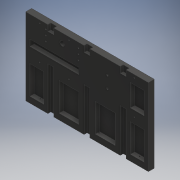
# Autodesk Inventor part: HB03
Saved by Autodesk Inventor 2017 (Build 210142000, 142)
## iProperties
Created: 2019-05-20
Part Number: HB03
Material: Polyethylene, High Density
Document SubType Name: Modeling
Designer: Dell
Density: 0.952 g/cm^3
Appearance: Smooth - Black
Mass: 3129.5 g
Surface Area: 4619.69 cm^2
Volume: 3287.29 cm^3
Author: Dell
Autodesk Inventor part; units mm, degrees
ref_plane "YZ Plane" through (0, 0, 0) normal (1, 0, 0) x (0, 1, 0)
ref_plane "XZ Plane" through (0, 0, 0) normal (0, 1, 0) x (-1, 0, 0)
ref_plane "XY Plane" through (0, 0, 0) normal (0, 0, 1) x (1, 0, 0)
sketch "Sketch1" plane through (0, 0, 0) normal (0, 0, 1) x (1, 0, 0)
  line L0 (0, 0) -> (525.78, 0)
  line L1 (525.78, 0) -> (525.78, 25.4)
  line L2 (525.78, 25.4) -> (0, 25.4)
  line L3 (0, 25.4) -> (0, 0)
  dimension "d0" = 525.78
  dimension "d1" = 25.4
  constraints: 8 end point, 2 parallel, 1 horizontal, 1 perpendicular
  measures "d0" distance of L2.end L1.end
  measures "d1" distance of L1.end L0.end
extrude "Extrusion1" add sketch "Sketch1" along normal blind 330.2
sketch "Sketch3" plane through (0, 25.4, 0) normal (0, 1, 0) x (1, 0, 0)
  line L0 (0, -330.2) -> (525.78, -330.2) construction
  line L1 (525.78, -330.2) -> (525.78, -241.3)
  line L2 (525.78, -241.3) -> (0, -241.3) construction
  line L3 (0, -241.3) -> (0, -330.2) construction
  line L4 (86.36, -308.25) -> (86.36, -263.25) construction
  circle A0 centre (86.36, -285.75) radius 2.3812
  circle A1 centre (86.36, -308.25) radius 2.3812
  circle A2 centre (86.36, -263.25) radius 2.3812
  line L5 (146.36, -280.75) -> (146.36, -300.75) construction
  line L6 (156.36, -263.25) -> (156.36, -308.25) construction
  line L7 (146.36, -300.75) -> (166.36, -300.75) construction
  line L8 (166.36, -280.75) -> (146.36, -280.75) construction
  line L9 (86.36, -263.25) -> (226.36, -263.25) construction
  line L10 (226.36, -308.25) -> (86.36, -308.25) construction
  line L11 (86.36, -285.75) -> (226.36, -285.75) construction
  line L12 (166.36, -300.75) -> (166.36, -280.75) construction
  line L13 (226.36, -263.25) -> (226.36, -308.25) construction
  circle A3 centre (226.36, -263.25) radius 2.3813
  circle A4 centre (226.36, -285.75) radius 2.3813
  circle A5 centre (226.36, -308.25) radius 2.3813
  circle A6 centre (156.36, -290.75) radius 10
  line L14 (0, 0) -> (0, -330.2) projected
  point P0 (525.78, 0)
  point P1 (0, -285.75)
  point P2 (146.36, -290.75)
  point P3 (166.36, -290.75)
  dimension "d16" = 45
  dimension "d17" = 140
  dimension "d18" = 4.7625
  dimension "d19" = 4.7625
  dimension "d20" = 4.7625
  dimension "d21" = 4.7625
  dimension "d22" = 4.7625
  dimension "d23" = 4.7625
  dimension "d24" = 60
  dimension "d25" = 7.5
  dimension "d26" = 20
  dimension "d27" = 20
  dimension "d28" = 86.36
  dimension "d29" = 88.9
  constraints: 28 end point, 7 midpoint, 6 centre point, 6 parallel, 5 coincident, 3 horizontal alignment, 3 perpendicular, 2 point on line, 1 horizontal, 2 other
  measures "d16" distance of L13.start L13.end
  measures "d17" distance of L9.start L13.start
  measures "d18" diameter of A2
  measures "d19" diameter of A0
  measures "d20" diameter of A1
  measures "d21" diameter of A5
  measures "d22" diameter of A4
  measures "d23" diameter of A3
  measures "d24" distance from line of L11.end L12
  measures "d25" distance between parallel lines of L10 L7
  measures "d26" distance of L12.end L8.end
  measures "d27" distance of L8.end L7.start
  measures "d28" distance between parallel lines of L3 L4
  measures "d29" distance of L2.end L0.start
extrude "Extrusion3" cut sketch "Sketch3" against normal through all
sketch "Sketch6" plane through (0, 0, 0) normal (0, 0, -1) x (-1, 0, 0)
  line L0 (0, 0) -> (-525.78, 0) projected
  line L1 (0, 0) -> (-525.78, 0) projected
  line L2 (-275.59, 0) -> (-250.19, 0)
  line L3 (-250.19, 0) -> (-250.19, 12.7)
  line L4 (-250.19, 12.7) -> (-275.59, 12.7)
  line L5 (-275.59, 12.7) -> (-275.59, 0)
  line L6 (-430.79, 0) -> (-405.39, 0)
  line L7 (-405.39, 0) -> (-405.39, 12.7)
  line L8 (-405.39, 12.7) -> (-430.79, 12.7)
  line L9 (-430.79, 12.7) -> (-430.79, 0)
  line L10 (-120.39, 0) -> (-94.99, 0)
  line L11 (-94.99, 0) -> (-94.99, 12.7)
  line L12 (-94.99, 12.7) -> (-120.39, 12.7)
  line L13 (-120.39, 12.7) -> (-120.39, 0)
  line L14 (-120.39, 6.35) -> (-405.39, 6.35)
  point P0 (-262.89, 0)
  point P1 (-94.99, 6.35)
  point P2 (-262.89, 6.35)
  point P3 (-262.89, 0)
  dimension "d34" = 25.4
  dimension "d35" = 12.7
  dimension "d36" = 25.4
  dimension "d37" = 12.7
  dimension "d40" = 25.4
  dimension "d41" = 12.7
  dimension "d47" = 285
  constraints: 26 end point, 7 midpoint, 7 parallel, 3 horizontal, 3 perpendicular, 3 point on line, 1 horizontal alignment, 1 vertical alignment
  measures "d34" distance of L4.end L3.end
  measures "d35" distance of L3.end L2.end
  measures "d36" distance of L8.end L7.end
  measures "d37" distance of L7.end L6.end
  measures "d40" distance of L11.end L12.end
  measures "d41" distance of L10.end L11.end
  measures "d47" distance of L14.start L14.end
extrude "Extrusion5" cut sketch "Sketch6" against normal blind 185 contours L0 L13 L12 L11 | L0 L5 L14 L3 | L14 L5 L4 L3 | L0 L9 L8 L7
sketch "Sketch8" plane through (0, 0, 330.2) normal (0, 0, 1) x (1, 0, 0)
  line L0 (94.99, 0) -> (120.39, 0) projected
  line L1 (94.99, 12.7) -> (94.99, 0) projected
  line L2 (120.39, 12.7) -> (94.99, 12.7) projected
  line L3 (120.39, 0) -> (120.39, 12.7) projected
  line L4 (250.19, 0) -> (275.59, 0) projected
  line L5 (250.19, 12.7) -> (250.19, 0) projected
  line L6 (275.59, 12.7) -> (250.19, 12.7) projected
  line L7 (275.59, 0) -> (275.59, 12.7) projected
  line L8 (405.39, 0) -> (430.79, 0) projected
  line L9 (405.39, 12.7) -> (405.39, 0) projected
  line L10 (430.79, 12.7) -> (405.39, 12.7) projected
  line L11 (430.79, 0) -> (430.79, 12.7) projected
  point P0 (0, 0)
extrude "Extrusion6" cut sketch "Sketch8" against normal blind 25.4
sketch "Sketch11" plane through (0, 0, 0) normal (0, -1, 0) x (1, 0, 0)
  circle A0 centre (60.195, 317.5) radius 2
  circle A1 centre (185.29, 317.5) radius 2
  circle A2 centre (340.49, 317.5) radius 2
  circle A3 centre (465.585, 317.5) radius 2
  circle A4 centre (465.585, 172.3) radius 2
  circle A5 centre (340.49, 172.3) radius 2
  circle A6 centre (185.29, 172.3) radius 2
  circle A7 centre (60.195, 172.3) radius 2
  line L0 (0, 330.2) -> (94.99, 330.2) projected
  line L1 (120.39, 330.2) -> (250.19, 330.2) projected
  line L2 (275.59, 330.2) -> (405.39, 330.2) projected
  line L3 (430.79, 330.2) -> (525.78, 330.2) projected
  line L4 (120.39, 304.8) -> (94.99, 304.8) projected
  line L5 (94.99, 185) -> (120.39, 185) projected
  point P0 (0, 0)
  point P1 (185.29, 330.2)
  point P2 (340.49, 330.2)
  dimension "d57" = 4
  dimension "d58" = 4
  dimension "d59" = 4
  dimension "d60" = 4
  dimension "d61" = 4
  dimension "d62" = 4
  dimension "d63" = 4
  dimension "d64" = 4
  dimension "d65" = 12.7
  dimension "d66" = 12.7
  dimension "d69" = 60.195
  dimension "d70" = 60.195
  constraints: 8 centre point, 6 horizontal alignment, 6 vertical alignment, 2 midpoint
  measures "d57" diameter of A0
  measures "d58" diameter of A1
  measures "d59" diameter of A2
  measures "d60" diameter of A3
  measures "d61" diameter of A4
  measures "d62" diameter of A5
  measures "d63" diameter of A6
  measures "d64" diameter of A7
  measures "d65" distance from line of A0.centre L4
  measures "d66" distance from line of L5 A7.centre
  measures "d69" horizontal distance of L0.start A0.centre
  measures "d70" horizontal distance of L3.end A3.centre
extrude "Extrusion8" cut sketch "Sketch11" against normal through all contours A0 | A1 | A3 | A4 | A6 | A7
sketch "Sketch12" plane through (0, 25.4, 0) normal (0, 1, 0) x (1, 0, 0)
  circle A0 centre (60.195, -172.3) radius 2 projected
  circle A1 centre (185.29, -172.3) radius 2 projected
  circle A2 centre (465.585, -172.3) radius 2 projected
  circle A3 centre (465.585, -317.5) radius 2 projected
  circle A4 centre (185.29, -317.5) radius 2 projected
  circle A5 centre (60.195, -317.5) radius 2 projected
  circle A6 centre (60.195, -172.3) radius 2 projected
  circle A7 centre (60.195, -172.3) radius 6.5
  circle A8 centre (60.195, -317.5) radius 2 projected
  circle A9 centre (60.195, -317.5) radius 6.5
  circle A10 centre (185.29, -317.5) radius 2 projected
  circle A11 centre (185.29, -317.5) radius 6.5
  circle A12 centre (185.29, -172.3) radius 2 projected
  circle A13 centre (185.29, -172.3) radius 6.5
  circle A14 centre (465.585, -317.5) radius 6.5
  circle A15 centre (465.585, -172.3) radius 2 projected
  circle A16 centre (465.585, -172.3) radius 6.5
  point P0 (0, 0)
  dimension "d71" = 13
  dimension "d72" = 13
  dimension "d73" = 13
  dimension "d74" = 13
  dimension "d75" = 13
  dimension "d76" = 13
  constraints: 6 centre point, 6 coincident
  measures "d71" diameter of A7
  measures "d72" diameter of A9
  measures "d73" diameter of A11
  measures "d74" diameter of A13
  measures "d75" diameter of A14
  measures "d76" diameter of A16
extrude "Extrusion9" cut sketch "Sketch12" against normal blind 12.7 contours A0 | A1 | A2 | A3 | A4 | A5 | A7 | A9 | A11 | A13 | A14 | A16
sketch "Sketch13" plane through (0, 25.4, 0) normal (0, 1, 0) x (1, 0, 0)
  circle A0 centre (349.98, -219.9) radius 4
  circle A1 centre (349.98, -269.9) radius 4
  line L0 (525.78, 0) -> (525.78, -330.2) projected
  line L1 (525.78, -330.2) -> (0, -330.2) projected
  point P0 (0, 0)
  dimension "d86" = 8
  dimension "d87" = 8
  dimension "d88" = 175.8
  dimension "d89" = 60.3
  dimension "d90" = 50
  constraints: 2 centre point, 1 vertical alignment
  measures "d86" diameter of A1
  measures "d87" diameter of A0
  measures "d88" distance from line of L0 A1.centre
  measures "d89" distance from line of L1 A1.centre
  measures "d90" distance of A1.centre A0.centre
extrude "Extrusion10" cut sketch "Sketch13" against normal through all
sketch "Sketch14" plane through (0, 25.4, 0) normal (0, 1, 0) x (1, 0, 0)
  circle A0 centre (349.98, -219.9) radius 4 projected
  circle A1 centre (349.98, -269.9) radius 4 projected
  circle A2 centre (349.98, -219.9) radius 7.5
  circle A3 centre (349.98, -269.9) radius 7.5
  point P0 (0, 0)
  dimension "d93" = 15
  dimension "d94" = 15
  constraints: 2 centre point, 2 coincident
  measures "d93" diameter of A2
  measures "d94" diameter of A3
extrude "Extrusion11" cut sketch "Sketch14" against normal blind 12.7 contours A0 | A1 | A2 | A3
sketch "Sketch9" plane through (0, 0, 0) normal (0, -1, 0) x (1, 0, 0)
  line L0 (297.99, 146.9) -> (382.99, 146.9)
  line L1 (382.99, 146.9) -> (382.99, 25.4)
  line L2 (382.99, 25.4) -> (297.99, 25.4)
  line L3 (297.99, 25.4) -> (297.99, 146.9)
  line L4 (448.285, 25.4) -> (508.285, 25.4)
  line L5 (508.285, 25.4) -> (508.285, 146.9)
  line L6 (508.285, 146.9) -> (448.285, 146.9)
  line L7 (448.285, 146.9) -> (448.285, 25.4)
  line L8 (142.79, 25.4) -> (227.79, 25.4)
  line L9 (227.79, 25.4) -> (227.79, 146.9)
  line L10 (227.79, 146.9) -> (142.79, 146.9)
  line L11 (142.79, 146.9) -> (142.79, 25.4)
  line L12 (17.495, 25.4) -> (77.495, 25.4)
  line L13 (77.495, 25.4) -> (77.495, 146.9)
  line L14 (77.495, 146.9) -> (17.495, 146.9)
  line L15 (17.495, 146.9) -> (17.495, 25.4)
  line L16 (430.79, 330.2) -> (525.78, 330.2) projected
  line L17 (275.59, 330.2) -> (405.39, 330.2) projected
  line L18 (120.39, 0) -> (250.19, 0) projected
  line L19 (0, 0) -> (94.99, 0) projected
  line L20 (430.79, 0) -> (525.78, 0) projected
  circle A0 centre (86.36, 263.25) radius 2.3812 projected
  circle A1 centre (465.585, 172.3) radius 2 construction
  circle A2 centre (465.585, 317.5) radius 2 construction
  line L21 (508.285, 197.7) -> (448.285, 197.7)
  line L22 (448.285, 197.7) -> (448.285, 292.1)
  line L23 (448.285, 292.1) -> (508.285, 292.1)
  line L24 (508.285, 292.1) -> (508.285, 197.7)
  line L25 (382.99, 146.9) -> (297.99, 146.9)
  line L26 (297.99, 146.9) -> (297.99, 292.1)
  line L27 (297.99, 292.1) -> (382.99, 292.1)
  line L28 (382.99, 292.1) -> (382.99, 146.9)
  line L29 (227.79, 210.4) -> (17.495, 210.4)
  line L30 (17.495, 210.4) -> (17.495, 237.85)
  line L31 (17.495, 237.85) -> (227.79, 237.85)
  line L32 (227.79, 237.85) -> (227.79, 210.4)
  line L33 (94.99, 185) -> (120.39, 185) projected
  line L34 (448.285, 210.4) -> (382.99, 210.4)
  line L35 (382.99, 210.4) -> (382.99, 279.4)
  line L36 (382.99, 279.4) -> (448.285, 279.4)
  line L37 (448.285, 279.4) -> (448.285, 210.4)
  line L38 (430.79, 185) -> (405.39, 185) projected
  line L39 (405.39, 304.8) -> (430.79, 304.8) projected
  line L40 (227.79, 210.4) -> (297.99, 210.4)
  line L41 (297.99, 210.4) -> (297.99, 237.85)
  line L42 (297.99, 237.85) -> (227.79, 237.85)
  line L43 (227.79, 237.85) -> (227.79, 210.4)
  point P0 (478.285, 146.9)
  point P1 (478.285, 330.2)
  point P2 (340.49, 146.9)
  point P3 (340.49, 330.2)
  point P4 (185.29, 25.4)
  point P5 (185.29, 0)
  point P6 (47.495, 25.4)
  point P7 (47.495, 0)
  dimension "d48" = 60
  dimension "d49" = 60
  dimension "d50" = 85
  dimension "d51" = 85
  dimension "d53" = 25.4
  dimension "d79" = 25.4
  dimension "d80" = 25.4
  dimension "d81" = 25.4
  dimension "d82" = 25.4
  dimension "d83" = 25.4
  dimension "d84" = 25.4
  dimension "d85" = 25.4
  constraints: 72 end point, 18 parallel, 9 horizontal, 9 perpendicular, 9 point on line, 8 midpoint, 8 vertical alignment, 7 horizontal alignment, 2 coincident
  measures "d48" distance of L12.start L12.end
  measures "d49" distance of L4.start L4.end
  measures "d50" distance of L8.start L8.end
  measures "d51" distance of L1.end L2.end
  measures "d53" distance between parallel lines of L20 L4
  measures "d79" distance from line of L6 A1.centre
  measures "d80" distance between parallel lines of L33 L29
  measures "d81" distance from line of A0.centre L31
  measures "d82" distance from line of A1.centre L21
  measures "d83" distance from line of A2.centre L23
  measures "d84" distance between parallel lines of L38 L34
  measures "d85" distance between parallel lines of L39 L36
extrude "Extrusion7" cut sketch "Sketch9" against normal blind 19.05 contours L0 L1 L2 L3 | L29 L30 L31 L32 | L22 L23 L24 L21 | L7 L6 L5 L4 | L11 L10 L9 L8 | L15 L14 L13 L12 | A0
sketch "Sketch15" plane through (0, 0, 0) normal (0, 0, -1) x (-1, 0, 0)
  circle A0 centre (-137.795, 12.7) radius 2
  circle A1 centre (-224.3975, 12.7) radius 2
  line L0 (0, 25.4) -> (0, 0) projected
  line L1 (-525.78, 25.4) -> (0, 25.4) projected
  line L2 (-262.89, 25.4) -> (-262.89, -36.2644)
  circle A2 centre (-387.985, 12.7) radius 2
  circle A3 centre (-301.3825, 12.7) radius 2
  point P0 (0, 12.7)
  dimension "d97" = 4
  dimension "d98" = 4
  dimension "d99" = 86.6025
  dimension "d100" = 137.795
  constraints: 4 centre point, 2 end point, 2 horizontal alignment, 2 midpoint, 2 symmetric about line, 1 vertical, 2 other
  measures "d97" diameter of A0
  measures "d98" diameter of A1
  measures "d99" distance of A0.centre A1.centre
  measures "d100" distance from line of L0 A0.centre
extrude "Extrusion12" cut sketch "Sketch15" against normal blind 38.1
sketch "Sketch16" plane through (0, 0, 0) normal (0, 0, -1) x (-1, 0, 0)
  circle A0 centre (-50, 12.7) radius 2
  line L0 (0, 25.4) -> (0, 0) projected
  circle A1 centre (-475.78, 12.7) radius 2
  line L1 (-525.78, 0) -> (-525.78, 25.4) projected
  point P0 (0, 12.7)
  point P1 (-525.78, 12.7)
  dimension "d103" = 4
  dimension "d104" = 50
  dimension "d105" = 4
  dimension "d106" = 50
  constraints: 2 centre point, 2 horizontal alignment, 2 midpoint
  measures "d103" diameter of A0
  measures "d104" distance from line of L0 A0.centre
  measures "d105" diameter of A1
  measures "d106" distance from line of A1.centre L1
extrude "Extrusion13" cut sketch "Sketch16" against normal blind 38.1
body "Solid1"
